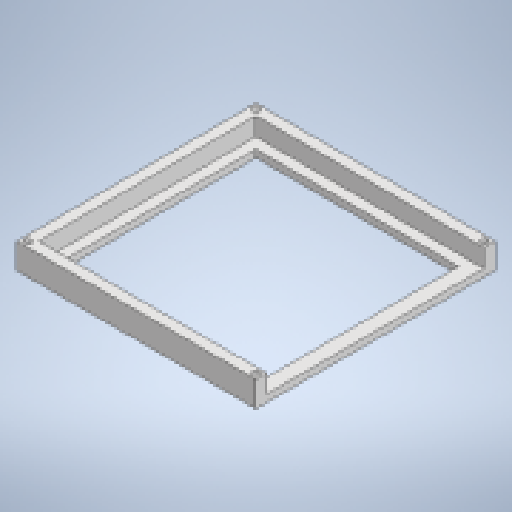
# Autodesk Inventor part: Disco_inferior
Saved by Autodesk Inventor 2024 (Build 280153000, 153)
## iProperties
Created: 2025-02-27
Part Number: Disco_inferior
Material: Genérico
Document SubType Name: Modeling
Designer: sergi
Density: 1 g/cm^3
Appearance: Valor por defecto
Author: sergi
Autodesk Inventor part; units mm, degrees
ref_plane "YZ Plane" through (0, 0, 0) normal (1, 0, 0) x (0, 1, 0)
ref_plane "XZ Plane" through (0, 0, 0) normal (0, 1, 0) x (-1, 0, 0)
ref_plane "XY Plane" through (0, 0, 0) normal (0, 0, 1) x (1, 0, 0)
sketch "Boceto1" plane through (0, 0, 0) normal (0, 1, 0) x (-1, 0, 0)
  line L0 (0, 0) -> (60, 0)
  line L1 (60, 0) -> (60, 60)
  line L2 (60, 60) -> (0, 60)
  line L3 (0, 60) -> (0, 0)
  line L4 (3, 57) -> (57, 57)
  line L5 (57, 57) -> (57, 3)
  line L6 (57, 3) -> (3, 3)
  line L7 (3, 3) -> (3, 57)
  line L8 (-3, 63) -> (63, 63)
  line L9 (63, 63) -> (63, -3)
  line L10 (63, -3) -> (-3, -3)
  line L11 (-3, -3) -> (-3, 63)
  dimension "d0" = 60
  dimension "d1" = 60
  dimension "d3" = 3
  dimension "d13" = 3
  constraints: 24 end point, 6 parallel, 3 perpendicular, 1 horizontal, 6 other
  measures "d0" distance of L2.end L1.end
  measures "d1" distance of L0.end L1.end
  measures "d3" distance between parallel lines of L2 L8
  measures "d13" distance between parallel lines of L2 L4
extrude "Extrusión1" add sketch "Boceto1" along normal blind 5 contours L8 L9 L10 L11
sketch "Boceto2" plane through (0, 0, 0) normal (0, -1, 0) x (1, 0, 0)
  line L0 (3, -3) -> (-63, -3) projected
  line L1 (3, 63) -> (3, -3) projected
  line L2 (-63, 63) -> (3, 63) projected
  line L3 (-63, -3) -> (-63, 63) projected
  line L4 (0, 0) -> (0, 60) projected
  line L5 (-60, 0) -> (0, 0) projected
  line L6 (-60, 60) -> (-60, 0) projected
  line L7 (0, 60) -> (-60, 60) projected
extrude "Extrusión2" add sketch "Boceto2" along normal blind 2 contours L0 L3 L2 L1 | L5 L6 L7 L4
sketch "Boceto3" plane through (0, 5, 0) normal (0, 1, 0) x (1, 0, 0)
  line L0 (0, 0) -> (0, -60) projected
  line L1 (0, -60) -> (3, -60)
  line L2 (3, -60) -> (3, 0)
  line L3 (3, 0) -> (0, 0)
  line L4 (0, 0) -> (0, -60)
  constraints: 8 end point, 2 parallel, 1 horizontal, 1 perpendicular
extrude "Extrusión3" cut sketch "Boceto3" against normal up to surface (5 mm away)
sketch "Boceto4" plane through (0, 0, 0) normal (0, 1, 0) x (1, 0, 0)
  line L0 (-60, 0) -> (3, 0) projected
  line L1 (-60, -60) -> (-60, 0) projected
  line L2 (-60, -60) -> (3, -60) projected
  line L3 (2, -60) -> (0, -60)
  line L4 (-1, -57) -> (-57, -57)
  line L5 (-57, -57) -> (-57, -3)
  line L6 (-57, -3) -> (-1, -3)
  line L7 (-1, -3) -> (-1, -57)
  line L8 (3, 0) -> (3, -60) projected
  point P0 (0, 0)
  dimension "d10" = 3
  constraints: 10 end point, 1 point on line, 2 other
  measures "d10" distance between parallel lines of L2 L4
extrude "Extrusión4" cut sketch "Boceto4" against normal blind 10 contours L4 L5 L6 L7
sketch "Boceto5" plane through (0, 5, 0) normal (0, 1, 0) x (1, 0, 0)
  line L0 (-60, 0) -> (3, 0) projected
  line L1 (3, 0) -> (3, 3) projected
  line L2 (3, 3) -> (-63, 3) projected
  line L3 (-63, 3) -> (-63, -63) projected
  line L4 (-63, -63) -> (3, -63) projected
  line L5 (3, -63) -> (3, -60) projected
  line L6 (3, -60) -> (-60, -60) projected
  line L7 (-60, -60) -> (-60, 0) projected
  line L8 (-60, -60) -> (-63, -63)
  circle A0 centre (-61.5, -61.5) radius 0.95
  line L9 (-60, 0) -> (-63, 3)
  circle A1 centre (-61.5, 1.5) radius 0.95
  line L10 (0, 0) -> (2.923, 2.923)
  line L11 (0, -60) -> (3, -63)
  circle A2 centre (1.5, -61.5) radius 0.95
  circle A3 centre (1.4615, 1.4615) radius 0.95
  point P0 (-61.5, 1.5)
  dimension "d14" = 1.9
  dimension "d16" = 1.9
  dimension "d18" = 1.9
  dimension "d20" = 1.9
  constraints: 8 end point, 4 centre point, 4 midpoint, 1 coincident, 1 point on line
  measures "d14" diameter of A0
  measures "d16" diameter of A1
  measures "d18" diameter of A2
  measures "d20" diameter of A3
hole "Agujero1" at (1.5, 5, 61.5) at (1.4615, 5, -1.4615) at (-61.5, 5, -1.5) at (-61.5, 5, 61.5) direction (0, -1, 0) diameter 1.9 end through all
